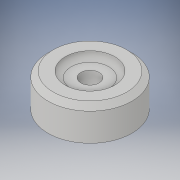
# Autodesk Inventor part: Diaphragme
Saved by Autodesk Inventor 2018 (Build 220112000, 112)
## iProperties
Created: 2020-03-27
Part Number: Diaphragme
Material: Generic
Document SubType Name: Modeling
Designer: emile
Density: 1 g/cm^3
Appearance: Default
Author: emile
Autodesk Inventor part; units mm, degrees
ref_plane "YZ Plane" through (0, 0, 0) normal (1, 0, 0) x (0, 1, 0)
ref_plane "XZ Plane" through (0, 0, 0) normal (0, 1, 0) x (-1, 0, 0)
ref_plane "XY Plane" through (0, 0, 0) normal (0, 0, 1) x (1, 0, 0)
sketch "Sketch1" plane through (0, 0, 0) normal (0, 0, 1) x (1, 0, 0)
  line L0 (0, 0) -> (0, 6.35)
  line L1 (12.7, 0) -> (0, 0)
  circle A0 centre (10.1178, 6.9428) radius 1.5875
  line L2 (0, 6.35) -> (8.6451, 6.35)
  line L3 (12.7, 0) -> (12.7, 6.35)
  line L4 (12.7, 6.35) -> (11.5905, 6.35)
  line L5 (9.525, 8.4155) -> (0, 8.4155)
  line L6 (0, 8.4155) -> (0, 6.35)
  line L7 (9.525, 8.4155) -> (11.5905, 6.35) construction
  line L8 (9.525, 8.4155) -> (9.525, 10.003)
  line L9 (9.525, 10.003) -> (0, 10.003)
  line L10 (0, 10.003) -> (0, 8.4155)
  line L11 (12.7, 6.35) -> (12.7, 10.003)
  line L12 (12.7, 10.003) -> (9.525, 10.003)
  dimension "d0" = 3.175
  dimension "d5" = 45
  dimension "d6" = 1.5875
  dimension "d7" = 3.175
  dimension "d8" = 6.35
  dimension "d14" = 2.921
  dimension "d37" = 12.7
  constraints: 26 end point, 6 perpendicular, 4 vertical, 3 point on circle, 2 horizontal, 1 centre point, 1 horizontal alignment
  measures "d0" diameter of A0
  measures "d5" angle of L4 L7
  measures "d6" distance of L5.start L8.end
  measures "d7" distance between parallel lines of L8 L3
  measures "d8" distance of L1.start L3.end
  measures "d14" distance of L5.start L4.end
  measures "d37" distance between parallel lines of L10 L11
revolve "Revolution1" add sketch "Sketch1" angle 360 about axis through (0, 10.003, 0) along (0, -1, 0)
sketch "Sketch8" plane through (0, 0, 0) normal (1, 0, 0) x (0, 1, 0)
  circle A0 centre (10.003, -5.734) radius 1.7653
  line L0 (10.003, 0) -> (8.2377, 0)
  line L1 (8.2377, 0) -> (8.2377, -5.734)
  line L2 (10.003, 13.6947) -> (10.003, -13.6947) projected
  line L3 (10.003, -5.734) -> (10.003, -3.9688) construction
  line L4 (-2.3537, 0) -> (14.1219, 0) projected
  point P0 (0, 0)
  dimension "d31" = 3.5306
  dimension "d32" = 3.9688
  constraints: 6 end point, 2 point on circle, 2 point on line, 1 centre point, 1 horizontal, 1 midpoint, 1 perpendicular, 1 tangent
  measures "d31" diameter of A0
  measures "d32" distance from line of L0 L3.end
revolve "Revolution3" cut sketch "Sketch8" angle 360 about axis through (0, -10, 0) along (0, 1, 0)
sketch "Sketch9" plane through (0, 8.2377, 0) normal (0, 1, 0) x (1, 0, 0)
  circle A0 centre (0, 0) radius 2.7781
  dimension "d34" = 5.5563
  constraints: 1 centre point, 1 coincident
  measures "d34" diameter of A0
extrude "Extrusion4" cut sketch "Sketch9" against normal through all
chamfer "Chamfer3" distance 1.5875 angle 45 1 edges at (-12.7, 10.003, 0)
body "Solid1"
